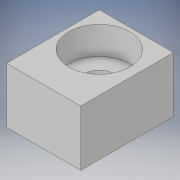
# Autodesk Inventor part: BoitCase
Saved by Autodesk Inventor 2019 (Build 230136000, 136)
## iProperties
Created: 2019-04-08
Part Number: BoitCase
Material: Generic
Document SubType Name: Modeling
Designer: Jorian Brusind
Density: 1 g/cm^3
Appearance: Default
Author: Jorian Brusind
Autodesk Inventor part; units mm, degrees
ref_plane "YZ Plane" through (0, 0, 0) normal (1, 0, 0) x (0, 1, 0)
ref_plane "XZ Plane" through (0, 0, 0) normal (0, 1, 0) x (-1, 0, 0)
ref_plane "XY Plane" through (0, 0, 0) normal (0, 0, 1) x (1, 0, 0)
sketch "Sketch1" plane through (0, 0, 0) normal (0, 1, 0) x (-1, 0, 0)
  line L0 (0, 0) -> (80, 0)
  line L1 (80, 0) -> (80, -100)
  line L2 (80, -100) -> (0, -100)
  line L3 (0, -100) -> (0, 0)
  dimension "d0" = 80
  dimension "d1" = 100
  constraints: 8 end point, 2 parallel, 1 horizontal, 1 perpendicular
  measures "d0" distance of L1.end L2.end
  measures "d1" distance of L0.end L1.end
extrude "Extrusion1" add sketch "Sketch1" along normal blind 60
sketch "Sketch2" plane through (0, 60, 0) normal (0, 1, 0) x (1, 0, 0)
  line L0 (-80, 100) -> (-80, 0) projected
  line L1 (-80, 0) -> (-43, 0)
  line L2 (-80, 0) -> (0, 0) projected
  line L3 (-43, 0) -> (-43, 63)
  circle A0 centre (-43, 63) radius 33
  line L4 (-43, 0) -> (-43, 15)
  dimension "d4" = 37
  dimension "d5" = 63
  dimension "d6" = 66
  constraints: 6 end point, 2 point on line, 1 centre point, 1 coincident, 1 perpendicular
  measures "d4" distance of L0.end L1.end
  measures "d5" distance of L1.end L3.end
  measures "d6" diameter of A0
extrude "Extrusion2" cut sketch "Sketch2" against normal blind 30
sketch "Sketch3" plane through (-43, 30, -63) normal (0, 1, 0) x (1, 0, 0)
  circle A0 centre (0, 0) radius 15
  line L0 (43, 37) -> (-37, 37) projected
  line L1 (-37, 37) -> (-37, -63) projected
  point P0 (43, -63)
  dimension "d11" = 30
  dimension "d12" = 37
  dimension "d13" = 37
  constraints: 1 centre point
  measures "d11" diameter of A0
  measures "d12" distance from line of L0 A0.centre
  measures "d13" distance from line of L1 A0.centre
extrude "Extrusion3" cut sketch "Sketch3" against normal blind 22
body "Solid1"
